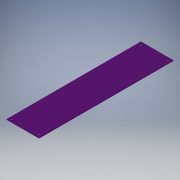
# Autodesk Inventor part: PRT1001-210 1U Board
Saved by Autodesk Inventor 2019 (Build 230136000, 136)
## iProperties
Created: 2019-07-02
Part Number: PRT1001-210 1U Board
Material: Generic
Document SubType Name: Modeling
Designer: james
Density: 1 g/cm^3
Appearance: Default(1)
Author: james
Autodesk Inventor part; units mm, degrees
ref_plane "YZ Plane" through (0, 0, 0) normal (1, 0, 0) x (0, 1, 0)
ref_plane "XZ Plane" through (0, 0, 0) normal (0, 1, 0) x (-1, 0, 0)
ref_plane "XY Plane" through (0, 0, 0) normal (0, 0, 1) x (1, 0, 0)
sketch "Sketch1" plane through (0, 0, 0) normal (0, 1, 0) x (-1, 0, 0)
  line L0 (10.6234, 96.3329) -> (-37.3766, 96.3329)
  line L1 (-37.3766, 96.3329) -> (-37.3766, -103.6671)
  line L2 (-37.3766, -103.6671) -> (10.6234, -103.6671)
  line L3 (10.6234, -103.6671) -> (10.6234, 96.3329)
  point P0 (0, 0)
  dimension "d0" = 200
  dimension "d1" = 48
  constraints: 8 end point, 2 parallel, 1 horizontal, 1 perpendicular
  measures "d0" distance of L0.end L1.end
  measures "d1" distance of L0.start L0.end
extrude "Extrusion1" add sketch "Sketch1" along normal blind 1
sketch "Sketch2" plane through (0, 1, 0) normal (0, 1, 0) x (1, 0, 0)
  line L0 (-10.6234, 103.6671) -> (-10.6234, -96.3329) projected
  line L1 (37.3766, -96.3329) -> (37.3766, 103.6671) projected
  line L2 (-10.6234, -96.3329) -> (37.3766, -96.3329) projected
  line L3 (37.3766, 103.6671) -> (-10.6234, 103.6671) projected
  point P0 (0, 0)
  point P1 (-6.6234, -92.3329)
  point P2 (33.3766, -92.3329)
  point P3 (33.3766, 99.6671)
  point P4 (-6.6234, 99.6671)
  dimension "d4" = 0
  dimension "d5" = 0
  dimension "d6" = 0
  dimension "d7" = 0
  dimension "d8" = 4
  dimension "d9" = 4
  dimension "d10" = 4
  dimension "d11" = 4
  measures "d4" vertical distance of point (33.377, 99.667) point (-6.623, 99.667)
  measures "d5" horizontal distance of point (33.377, -92.333) point (33.377, 99.667)
  measures "d6" horizontal distance of point (-6.623, -92.333) point (-6.623, 99.667)
  measures "d7" vertical distance of point (33.377, -92.333) point (-6.623, -92.333)
  measures "d8" distance from line of L0 point (-6.623, -92.333)
  measures "d9" distance from line of L1 point (33.377, -92.333)
  measures "d10" distance from line of L2 point (33.377, -92.333)
  measures "d11" distance from line of L3 point (33.377, 99.667)
hole "Hole1" at (-6.6234, 1, 92.3329) at (33.3766, 1, 92.3329) at (33.3766, 1, -99.6671) at (-6.6234, 1, -99.6671) direction (0, -1, 0) diameter 3 depth 25.4 tip angle 118.188
equation "\"d1\" = BoardWidth"
equation "\"d2\" = BoardHeight"
equation "\"d8\" = ScrewHoleOffset"
equation "\"d9\" = ScrewHoleOffset"
equation "\"d10\" = ScrewHoleOffset"
equation "\"d11\" = ScrewHoleOffset"
equation "\"d12\" = ScrewSize"
equation "\"BoardLength\" = 556"
equation "\"BoardWidth\" = 48"
equation "\"ScrewSize\" = 3"
equation "\"ScrewHoleOffset\" = 4"
equation "\"BoardGap\" = 4"
equation "\"BoardHeight\" = 1"
equation "\"HorizOffsetBetweenScrews\" = 192"
equation "\"BaseWidth\" = 556"
equation "\"BaseLength\" = 648"
equation "\"TwoBoardWidth\" = 444"
equation "\"NumberOfRows\" = 254"
equation "\"NumberOfGaps\" = 228.6"
body "Solid1"
